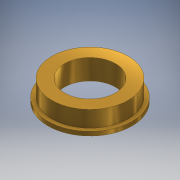
# Autodesk Inventor part: ベアリング　内径10
Saved by Autodesk Inventor 2016 (Build 200138000, 138)
## iProperties
Created: 2018-04-10
Part Number: ベアリング　内径10
Material: 一般
Document SubType Name: Modeling
Designer: Takumi
Mass: 2.1 g
Surface Area: 5.88499 cm^2
Volume: 0.422387 cm^3
Density: 4.97174 g/cm^3
Appearance: 真鍮 - つや出し
Author: Takumi
Autodesk Inventor part; units mm, degrees
ref_plane "YZ Plane" through (0, 0, 0) normal (1, 0, 0) x (0, 1, 0)
ref_plane "XZ Plane" through (0, 0, 0) normal (0, 1, 0) x (-1, 0, 0)
ref_plane "XY Plane" through (0, 0, 0) normal (0, 0, 1) x (1, 0, 0)
sketch "スケッチ1" plane through (0, 0, 0) normal (0, 0, 1) x (1, 0, 0)
  circle A0 centre (0, 0) radius 5
  circle A1 centre (0, 0) radius 7.5
  circle A2 centre (0, 0) radius 8.25
  dimension "d0" = 10
  dimension "d1" = 15
  dimension "d2" = 16.5
  constraints: 3 centre point, 3 coincident
  measures "d0" diameter of A0
  measures "d1" diameter of A1
  measures "d2" diameter of A2
extrude "押し出し1" add sketch "スケッチ1" along normal blind 3.2 contours A1
extrude "押し出し2" add sketch "スケッチ1" against normal blind 0.8 contours A1 | A2
